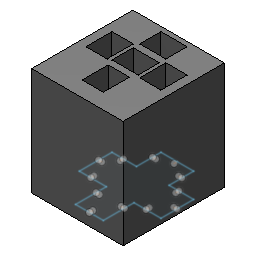
Кронштейн реле 1 (Autodesk Fusion 360 design; units mm, degrees)
Autodesk Fusion 360 part; units mm, degrees
sketch "Sketch1" plane through (0, 0, 0) normal (0, 0, 1) x (1, 0, 0)
  line L0 (0, 0) -> (150, 0)
  line L1 (150, 0) -> (150, 80)
  line L2 (150, 80) -> (0, 80)
  line L3 (0, 80) -> (0, 0)
  line L4 (0, 40) -> (150, 40) construction
  line L5 (75, 80) -> (75, 0) construction
  line L6 (145, 0) -> (145, 3) construction
  line L7 (145, 3) -> (0, 3) construction
  line L8 (150, 10.0271) -> (147, 10.0271) construction
  line L9 (147, 10.0271) -> (147, 80) construction
  line L10 (143.7923, 80) -> (143.7923, 77) construction
  line L11 (143.7923, 77) -> (0, 77) construction
  line L12 (0, 74) -> (3, 74) construction
  line L13 (3, 74) -> (3, 0) construction
  line L14 (147, 77) -> (146, 77) construction
  line L15 (146, 77) -> (146, 0) construction
  line L16 (146, 77) -> (146, 76) construction
  line L17 (146, 76) -> (0, 76) construction
  line L18 (3, 76) -> (4, 76) construction
  line L19 (4, 76) -> (4, 0) construction
  line L20 (4, 3) -> (4, 4) construction
  line L21 (4, 4) -> (146, 4) construction
  line L22 (146, 76) -> (118, 76)
  line L23 (118, 76) -> (118, 45)
  line L24 (118, 45) -> (146, 45)
  line L25 (146, 45) -> (146, 76)
  line L26 (146, 4) -> (118, 4)
  line L27 (118, 4) -> (118, 35)
  line L28 (118, 35) -> (146, 35)
  line L29 (146, 35) -> (146, 4)
  line L30 (118, 64) -> (113, 64) construction
  line L31 (113, 76) -> (85, 76)
  line L32 (85, 76) -> (85, 45)
  line L33 (85, 45) -> (113, 45)
  line L34 (113, 45) -> (113, 76)
  line L35 (118, 19.5) -> (113, 19.5) construction
  line L36 (85, 4) -> (113, 4)
  line L37 (113, 4) -> (113, 35)
  line L38 (113, 35) -> (85, 35)
  line L39 (85, 35) -> (85, 4)
  line L40 (146, 60.5) -> (132, 60.5) construction
  line L41 (132, 60.5) -> (132, 45) construction
  line L42 (132, 60.5) -> (118, 60.5) construction
  line L43 (132, 60.5) -> (132, 76) construction
  line L44 (134.1559, 76) -> (134.1559, 74.6) construction
  line L45 (132, 74.6) -> (128, 74.6)
  line L46 (128, 74.6) -> (128, 68.1)
  line L47 (128, 68.1) -> (136, 68.1)
  line L48 (136, 68.1) -> (136, 74.6)
  line L49 (136, 74.6) -> (132, 74.6)
  line L50 (132, 68.1) -> (132, 57.7) construction
  line L51 (132, 57.7) -> (135.25, 57.7)
  line L52 (135.25, 57.7) -> (135.25, 49.7)
  line L53 (135.25, 49.7) -> (128.75, 49.7)
  line L54 (128.75, 49.7) -> (128.75, 57.7)
  line L55 (128.75, 57.7) -> (132, 57.7)
  line L56 (136, 69.6047) -> (137, 69.6047) construction
  line L57 (136, 68.1) -> (136, 67.1) construction
  line L58 (137, 67.1) -> (143.5, 67.1)
  line L59 (143.5, 67.1) -> (143.5, 59.1)
  line L60 (143.5, 59.1) -> (137, 59.1)
  line L61 (137, 59.1) -> (137, 67.1)
  line L62 (128, 68.1) -> (128, 67.1) construction
  line L63 (128, 67.1) -> (127, 67.1) construction
  line L64 (127, 67.1) -> (120.5, 67.1)
  line L65 (120.5, 67.1) -> (120.5, 59.1)
  line L66 (120.5, 59.1) -> (127, 59.1)
  line L67 (127, 59.1) -> (127, 67.1)
  line L68 (133.5018, 68.1) -> (133.5018, 66.1) construction
  line L69 (136, 66.1) -> (128, 66.1)
  line L70 (128, 66.1) -> (128, 59.6)
  line L71 (128, 59.6) -> (136, 59.6)
  line L72 (136, 59.6) -> (136, 66.1)
  dimension "d1" = 150
  dimension "d2" = 80
  dimension "d3" = 3
  dimension "d4" = 3
  dimension "d5" = 3
  dimension "d6" = 3
  dimension "d7" = 1
  dimension "d8" = 1
  dimension "d9" = 1
  dimension "d10" = 1
  dimension "d11" = 28
  dimension "d12" = 31
  dimension "d13" = 28
  dimension "d14" = 31
  dimension "d15" = 5
  dimension "d16" = 28
  dimension "d17" = 31
  dimension "d18" = 5
  dimension "d21" = 1.4
  dimension "d22" = 4
  dimension "d23" = 6.5
  dimension "d24" = 8
  dimension "d25" = 10.4
  dimension "d26" = 3.25
  dimension "d27" = 8
  dimension "d28" = 6.5
  dimension "d29" = 1
  dimension "d30" = 1
  dimension "d31" = 6.5
  dimension "d32" = 8
  dimension "d33" = 6.5
  dimension "d34" = 6.5
  dimension "d35" = 8
  dimension "d51" = 2
  dimension "d52" = 6.5
  dimension "d53" = 8
  constraint horizontal L0
  constraint vertical L1
  constraint horizontal L2
  constraint vertical L3
  constraint coincident L0.start L3.end
  constraint midpoint L3 L4.start
  constraint midpoint L1 L4.end
  constraint midpoint L2 L5.start
  constraint midpoint L0 L5.end
  constraint coincident L0 L6.start
  constraint perpendicular L0 L6
  constraint coincident L3 L7.end
  constraint perpendicular L3 L7
  constraint coincident L1 L8.start
  constraint perpendicular L1 L8
  constraint coincident L2 L9.end
  constraint perpendicular L2 L9
  constraint coincident L2 L10.start
  constraint perpendicular L2 L10
  constraint coincident L3 L11.end
  constraint perpendicular L3 L11
  constraint coincident L3 L12.start
  constraint perpendicular L3 L12
  constraint coincident L0 L13.end
  constraint perpendicular L0 L13
  constraint coincident L9 L14.start
  constraint perpendicular L10 L14
  constraint coincident L0 L15.end
  constraint perpendicular L0 L15
  constraint coincident L15 L16.end
  constraint coincident L3 L17.end
  constraint perpendicular L3 L17
  constraint coincident L17 L18.start
  constraint coincident L17 L18.end
  constraint coincident L0 L19.end
  constraint perpendicular L0 L19
  constraint coincident L19 L20.start
  constraint coincident L7 L20.start
  constraint coincident L19 L20.end
  constraint coincident L15 L21.end
  constraint perpendicular L15 L21
  constraint coincident L17 L22.end
  constraint perpendicular L17 L23
  constraint coincident L15 L24.end
  constraint perpendicular L15 L24
  constraint coincident L21 L26.end
  constraint perpendicular L21 L27
  constraint coincident L15 L28.end
  constraint perpendicular L15 L28
  constraint coincident L23 L30.start
  constraint perpendicular L23 L30
  constraint coincident L17 L31.start
  constraint coincident L17 L31.end
  constraint perpendicular L17 L32
  constraint perpendicular L32 L33
  constraint perpendicular L17 L34
  constraint midpoint L27 L35.start
  constraint perpendicular L27 L35
  constraint coincident L21 L36.start
  constraint coincident L21 L36.end
  constraint perpendicular L4 L37
  constraint perpendicular L21 L39
  constraint midpoint L25 L40.start
  constraint perpendicular L25 L40
  constraint midpoint L24 L41.end
  constraint perpendicular L24 L41
  constraint midpoint L23 L42.end
  constraint midpoint L22 L43.end
  constraint coincident L22 L44.start
  constraint perpendicular L22 L44
  constraint coincident L43 L45.start
  constraint perpendicular L43 L45
  constraint perpendicular L22 L46
  constraint perpendicular L43 L47
  constraint perpendicular L22 L48
  constraint perpendicular L43 L49
  constraint midpoint L47 L50.start
  constraint perpendicular L47 L50
  constraint perpendicular L23 L51
  constraint perpendicular L51 L52
  constraint perpendicular L41 L53
  constraint perpendicular L51 L54
  constraint perpendicular L41 L55
  constraint coincident L48 L56.start
  constraint perpendicular L48 L56
  constraint perpendicular L47 L57
  constraint perpendicular L57 L58
  constraint perpendicular L40 L59
  constraint perpendicular L59 L60
  constraint perpendicular L47 L62
  constraint perpendicular L62 L63
  constraint perpendicular L46 L64
  constraint perpendicular L42 L65
  constraint perpendicular L65 L66
  constraint perpendicular L63 L67
  constraint coincident L47 L68.start
  constraint perpendicular L47 L68
  constraint perpendicular L43 L69
  constraint perpendicular L42 L70
  constraint perpendicular L41 L71
  measures "d1" distance of L0.start L0.end
  measures "d2" distance of L0.start L2.end
  measures "d3" distance of L6.start L6.end
  measures "d4" distance of L8.start L8.end
  measures "d5" distance of L10.start L10.end
  measures "d6" distance of L12.start L12.end
  measures "d7" distance of L14.start L14.end
  measures "d8" distance of L14.end L16.end
  measures "d9" distance of L18.start L18.end
  measures "d10" distance of L20.start L20.end
  measures "d11" distance of L16.end L22.end
  measures "d12" distance of L22.end L23.end
  measures "d13" distance of L21.end L26.end
  measures "d14" distance of L26.end L27.end
  measures "d15" distance of L30.start L30.end
  measures "d16" distance of L31.start L31.end
  measures "d17" distance of L31.end L32.end
  measures "d18" distance of L35.start L35.end
  measures "d21" distance of L44.start L44.end
  measures "d22" distance of L45.start L45.end
  measures "d23" distance of L45.end L46.end
  measures "d24" distance of L46.end L47.end
  measures "d25" distance of L50.start L50.end
  measures "d26" distance of L50.end L51.end
  measures "d27" distance of L51.end L52.end
  measures "d28" distance of L52.end L53.end
  measures "d29" distance of L56.start L56.end
  measures "d30" distance of L47.end L57.end
  measures "d31" distance of L58.start L58.end
  measures "d32" distance of L58.end L59.end
  measures "d33" distance of L59.end L60.end
  measures "d34" distance of L63.end L64.end
  measures "d35" distance of L64.end L65.end
  measures "d51" distance of L68.start L68.end
  measures "d52" distance of L69.end L70.end
  measures "d53" distance of L70.end L71.end
extrude "Extrude1" add sketch "Sketch1" along normal blind 35 contours L0 L1 L2 L3 | L22 L23 L24 L25 | L26 L27 L28 L29 | L31 L32 L33 L34 | L36 L37 L38 L39 | L45 L46 L47 L48 L49 | L51 L52 L53 L54 L55 | L58 L59 L60 L61 | L64 L65 L66 L67 | L69 L70 L71 L72 makes body 1
shell "Shell1" thickness 2 removed faces 1 at (50, 53.3333, 0) on bodies 1
extrude "Extrude2" add sketch "Sketch1" along normal blind 33 separate body contours L22 L23 L24 L25 makes body 2
sketch "Sketch3" plane through (0, 0, 0) normal (0, 0, 1) x (1, 0, 0)
  line L0 (132, 74.6) -> (132, 75.6) construction
  line L1 (128, 73) -> (127, 73) construction
  line L2 (123, 67.1) -> (123, 68.1) construction
  line L3 (120.5, 64) -> (119.5, 64) construction
  line L4 (123, 59.1) -> (123, 58.1) construction
  line L5 (128.75, 54.95) -> (127.75, 54.95) construction
  line L6 (132, 49.7) -> (132, 48.7) construction
  line L7 (135.25, 55.15) -> (136.25, 55.15) construction
  line L8 (139.9, 59.1) -> (139.9, 58.1) construction
  line L9 (143.5, 63) -> (144.5, 63) construction
  line L10 (140, 67.1) -> (140, 68.1) construction
  line L11 (136, 72) -> (137, 72) construction
  line L12 (132, 75.6) -> (127, 75.6)
  line L13 (127, 75.6) -> (127, 68.1)
  line L14 (127, 68.1) -> (119.5, 68.1)
  line L15 (119.5, 68.1) -> (119.5, 58.1)
  line L16 (119.5, 58.1) -> (127.75, 58.1)
  line L17 (127.75, 58.1) -> (127.75, 48.7)
  line L18 (127.75, 48.7) -> (136.25, 48.7)
  line L19 (136.25, 48.7) -> (136.25, 58.1)
  line L20 (136.25, 58.1) -> (144.5, 58.1)
  line L21 (144.5, 58.1) -> (144.5, 68.1)
  line L22 (144.5, 68.1) -> (137, 68.1)
  line L23 (137, 68.1) -> (137, 75.6)
  line L24 (137, 75.6) -> (132, 75.6)
  dimension "d39" = 1
  dimension "d40" = 1
  dimension "d41" = 1
  dimension "d42" = 1
  dimension "d43" = 1
  dimension "d44" = 1
  dimension "d45" = 1
  dimension "d46" = 1
  dimension "d47" = 1
  dimension "d48" = 1
  dimension "d49" = 1
  dimension "d50" = 1
  constraint vertical L0
  constraint horizontal L1
  constraint perpendicular L1 L2
  constraint horizontal L3
  constraint vertical L4
  constraint horizontal L5
  constraint vertical L6
  constraint horizontal L7
  constraint vertical L8
  constraint horizontal L9
  constraint vertical L10
  constraint horizontal L11
  constraint perpendicular L0 L12
  constraint perpendicular L1 L13
  constraint perpendicular L2 L14
  constraint perpendicular L14 L15
  constraint perpendicular L15 L16
  constraint perpendicular L5 L17
  constraint perpendicular L17 L18
  constraint perpendicular L18 L19
  constraint perpendicular L19 L20
  constraint perpendicular L20 L21
  constraint perpendicular L21 L22
  constraint perpendicular L12 L23
  constraint perpendicular L0 L24
  measures "d39" distance of L0.start L0.end
  measures "d40" distance of L1.start L1.end
  measures "d41" distance of L2.start L2.end
  measures "d42" distance of L3.start L3.end
  measures "d43" distance of L4.start L4.end
  measures "d44" distance of L5.start L5.end
  measures "d45" distance of L6.start L6.end
  measures "d46" distance of L7.start L7.end
  measures "d47" distance of L8.start L8.end
  measures "d48" distance of L9.start L9.end
  measures "d49" distance of L10.start L10.end
  measures "d50" distance of L11.start L11.end
sketch "Sketch4" plane through (0, 0, 0) normal (0, 0, 1) x (1, 0, 0)
copy_body "CopyPasteBodies1" bodies 2 makes body 3
move_body "Move1" bodies 3 to x (1, 0, 0) y (0, 1, 0) z (0, 0, 1) at (-33, 0, 0)
copy_body "CopyPasteBodies2" bodies 2 makes body 4
move_body "Move2" bodies 4 to x (1, 0, 0) y (0, 1, 0) z (0, 0, 1) at (0, -41, 0)
copy_body "CopyPasteBodies3" bodies 2 makes body 5
move_body "Move3" bodies 5 to x (1, 0, 0) y (0, 1, 0) z (0, 0, 1) at (-33, -41, 0)
copy_body "CopyPasteBodies5" bodies 3 makes body 6
move_body "Move4" bodies 6 to x (1, 0, 0) y (0, 1, 0) z (0, 0, 1) at (-33, 0, 0)
copy_body "CopyPasteBodies6" bodies 5 makes body 7
move_body "Move5" bodies 7 to x (1, 0, 0) y (0, 1, 0) z (0, 0, 1) at (-33, 0, 0)
copy_body "CopyPasteBodies7" bodies 7 makes body 8
move_body "Move6" bodies 8 to x (1, 0, 0) y (0, 1, 0) z (0, 0, 1) at (-33, 0, 0)
copy_body "CopyPasteBodies8" bodies 6 makes body 9
move_body "Move7" bodies 9 to x (1, 0, 0) y (0, 1, 0) z (0, 0, 1) at (-33, 0, 0)
hidden bodies 1 3 4 5 6 7 8 9
